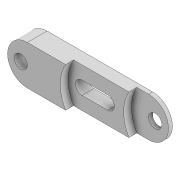
# Autodesk Inventor part: GripP4
Saved by Autodesk Inventor 2021 (Build 250183000, 183)
## iProperties
Created: 2022-09-30
Part Number: GripP4
Material: Generic
Document SubType Name: Modeling
Designer: brian
Density: 1 g/cm^3
Appearance: Default
Mass: 26.7147 g
Surface Area: 94.5739 cm^2
Volume: 26.7147 cm^3
Author: brian
Autodesk Inventor part; units mm, degrees
ref_plane "YZ Plane" through (0, 0, 0) normal (1, 0, 0) x (0, 1, 0)
ref_plane "XZ Plane" through (0, 0, 0) normal (0, 1, 0) x (-1, 0, 0)
ref_plane "XY Plane" through (0, 0, 0) normal (0, 0, 1) x (1, 0, 0)
sketch "Sketch1" plane through (0, 0, 0) normal (0, 0, 1) x (1, 0, 0)
  line L0 (15, 0) -> (95, 0)
  line L1 (110, 15) -> (110, 15)
  line L2 (95, 30) -> (15, 30)
  line L3 (0, 15) -> (0, 15)
  circle A0 centre (10, 15) radius 5
  circle A1 centre (100, 15) radius 5
  arc A2 (110, 15) -> (95, 30) centre (95, 15) ccw
  arc A3 (95, 0) -> (110, 15) centre (95, 15) ccw
  arc A4 (0, 15) -> (15, 0) centre (15, 15) ccw
  arc A5 (15, 30) -> (0, 15) centre (15, 15) ccw
  point P0 (0, 0)
  point P1 (110, 0)
  point P2 (110, 30)
  point P3 (0, 15)
  dimension "d1" = 30
  dimension "d14" = 10
  dimension "d15" = 10
  dimension "d16" = 10
  dimension "d17" = 90
  dimension "d18" = 15
  dimension "d21" = 15
  constraints: 8 end point, 8 point on circle, 8 tangent, 6 centre point, 6 point on line, 4 equal radius, 2 parallel, 1 horizontal, 1 perpendicular
  measures "d1" distance of point (110, 0) point (110, 30)
  measures "d14" diameter of A0
  measures "d15" distance from line of L3 A0.centre
  measures "d16" distance from line of A1.centre L1
  measures "d17" distance of A1.centre A0.centre
  measures "d18" radius of A2
  measures "d21" distance from line of L2 A1.centre
extrude "Extrusion1" add sketch "Sketch1" along normal blind 3
sketch "Sketch2" plane through (0, 0, 3) normal (0, 0, 1) x (1, 0, 0)
  arc A0 (95, 0) -> (95, 30) centre (95, 15) ccw projected
  line L0 (95, 30) -> (15, 30) projected
  arc A1 (15, 30) -> (15, 0) centre (15, 15) ccw projected
  line L1 (15, 0) -> (95, 0) projected
  circle A2 centre (100, 15) radius 5 projected
  circle A3 centre (10, 15) radius 5 projected
  circle A4 centre (100, 15) radius 5 projected
  line L2 (15, 0) -> (95, 0) projected
  line L3 (95, 30) -> (15, 30) projected
  circle A5 centre (112, 15) radius 30
  point P0 (0, 0)
  point P1 (86.0192, 0)
  point P2 (86.0192, 30)
  dimension "d32" = 60
  dimension "d33" = 12
  constraints: 1 centre point, 1 horizontal alignment
  measures "d32" diameter of A5
  measures "d33" distance of A2.centre A5.centre
extrude "Extrusion2" add sketch "Sketch2" along normal blind 6 contours L1 A1 L0 A5
sketch "Sketch3" plane through (0, 0, 0) normal (0, 0, -1) x (-1, 0, 0)
  arc A0 (-95, 30) -> (-95, 0) centre (-95, 15) ccw projected
  line L0 (-15, 0) -> (-95, 0) projected
  arc A1 (-15, 0) -> (-15, 30) centre (-15, 15) ccw projected
  line L1 (-95, 30) -> (-15, 30) projected
  circle A2 centre (-100, 15) radius 5 projected
  circle A3 centre (-10, 15) radius 5 projected
  circle A4 centre (-50.5, 15) radius 5
  circle A5 centre (-70, 15) radius 5
  circle A6 centre (-10, 15) radius 5 projected
  line L2 (-50.5, 20) -> (-70, 20)
  line L3 (-70, 10) -> (-50.5, 10)
  point P0 (0, 0)
  dimension "d26" = 40.5
  dimension "d27" = 30
  dimension "d28" = 10
  constraints: 4 end point, 4 point on circle, 2 centre point, 2 equal radius, 2 horizontal alignment, 2 tangent
  measures "d26" distance of A3.centre A4.centre
  measures "d27" distance of A2.centre A5.centre
  measures "d28" diameter of A3
extrude "Extrusion3" cut sketch "Sketch3" against normal up to surface (9 mm away) contours A4 | A4 L3 A5 L2 | A5
sketch "Sketch4" plane through (0, 0, 9) normal (0, 0, 1) x (1, 0, 0)
  line L0 (70, 10) -> (50.5, 10) projected
  arc A0 (50.5, 20) -> (50.5, 10) centre (50.5, 15) ccw projected
  line L1 (50.5, 20) -> (70, 20) projected
  arc A1 (70, 10) -> (70, 20) centre (70, 15) ccw projected
  line L2 (15, 0) -> (86.0192, 0) projected
  arc A2 (86.0192, 30) -> (86.0192, 0) centre (112, 15) ccw projected
  line L3 (86.0192, 30) -> (15, 30) projected
  arc A3 (15, 30) -> (15, 0) centre (15, 15) ccw projected
  circle A4 centre (10, 15) radius 5 projected
  circle A5 centre (70, 15) radius 15
  line L4 (15, 0) -> (95, 0) projected
  circle A6 centre (70, 15) radius 30
  point P0 (0, 0)
  point P1 (44.0192, 0)
  point P2 (44.0192, 30)
  dimension "d34" = 60
  dimension "d35" = 60
  constraints: 2 centre point, 1 coincident, 1 horizontal alignment, 1 tangent
  measures "d34" distance of A4.centre A5.centre
  measures "d35" diameter of A6
extrude "Extrusion4" add sketch "Sketch4" along normal blind 6 contours L2 A3 L3 A6
sketch "Sketch5" plane through (0, 0, 0) normal (0, 0, -1) x (-1, 0, 0)
  circle A0 centre (-30.25, 15) radius 2.5
  arc A1 (-50.5, 10) -> (-50.5, 20) centre (-50.5, 15) ccw projected
  circle A2 centre (-10, 15) radius 5 projected
  point P0 (0, 0)
  dimension "d38" = 5
  dimension "d39" = 40.5
  dimension "d40" = 20.25
  constraints: 1 centre point, 1 horizontal alignment
  measures "d38" diameter of A0
  measures "d39" distance of A1.centre A2.centre
  measures "d40" distance of A1.centre A0.centre
extrude "Extrusion5" cut sketch "Sketch5" against normal blind 0.1 contours A0
equation "\"d1\" = d0"
equation "\"d14\" = d6"
equation "\"d15\" = d14"
equation "\"d16\" = d15"
equation "\"d18\" = 0.5 * d1"
equation "\"d21\" = 0.5 * d1"
equation "\"d19\" = d11"
equation "\"d32\" = 2 * d0"
equation "\"d33\" = 0.4 * d0"
equation "\"d22\" = 2 * d11"
equation "\"d26\" = 1.35 * d0"
equation "\"d27\" = d0"
equation "\"d34\" = 2 * d0"
equation "\"d35\" = 2 * d0"
equation "\"d36\" = 2 * d11"
equation "\"d40\" = 0.5 * d39"
equation "\"d6\" = 10"
equation "\"d11\" = 3"
equation "\"d0\" = 30"
body "Solid1"
